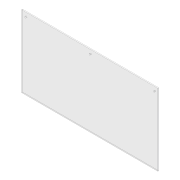
# Autodesk Inventor part: FE-00008
Saved by Autodesk Inventor 2012 (Build 160160000, 160)
## iProperties
Created: 2008-06-02
Part Number: FE-00008
Document SubType Name: Modeling
Designer: mcyr
Density: 1 g/cm^3
Description: Field Plastic "A"
Mass: 2800.83 g
Surface Area: 9004.63 cm^2
Volume: 2800.83 cm^3
Material: Default
Title: FE-00008
Author: mcyr
Autodesk Inventor part; units mm, degrees
ref_plane "YZ Plane" through (0, 0, 0) normal (1, 0, 0) x (0, 1, 0)
ref_plane "XZ Plane" through (0, 0, 0) normal (0, 1, 0) x (-1, 0, 0)
ref_plane "XY Plane" through (0, 0, 0) normal (0, 0, 1) x (1, 0, 0)
sketch "Sketch1" plane through (0, 0, 0) normal (0, 0, 1) x (1, 0, 0)
  line L0 (-44.592, 0) -> (869.808, 0)
  line L1 (869.808, 482.6) -> (-44.592, 482.6)
  line L2 (-44.592, 482.6) -> (-44.592, 0)
  line L3 (869.808, 0) -> (869.808, 482.6)
  circle A0 centre (-19.192, 450.85) radius 4.7625
  circle A1 centre (412.608, 450.85) radius 4.7625
  circle A2 centre (844.408, 450.85) radius 4.7625
  dimension "d0" = 914.4
  dimension "d1" = 482.6
  dimension "d2" = 9.525
  dimension "d3" = 9.525
  dimension "d4" = 9.525
  dimension "d5" = 31.75
  dimension "d6" = 31.75
  dimension "d7" = 31.75
  dimension "d8" = 25.4
  dimension "d9" = 457.2
  dimension "d10" = 889
  constraints: 8 end point, 3 centre point, 2 parallel, 1 horizontal, 1 perpendicular
  measures "d0" distance of L0.start L0.end
  measures "d1" distance of L1.end L0.start
  measures "d2" diameter of A0
  measures "d3" diameter of A1
  measures "d4" diameter of A2
  measures "d5" vertical distance of L1.end A0.centre
  measures "d6" distance from line of L1 A1.centre
  measures "d7" distance from line of L1 A2.centre
  measures "d8" horizontal distance of A0.centre L1.end
  measures "d9" horizontal distance of A1.centre L1.end
  measures "d10" horizontal distance of A2.centre L1.end
extrude "Extrusion1" add sketch "Sketch1" along normal blind 6.35
body "Solid1"
